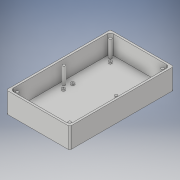
# Autodesk Inventor part: Box
Saved by Autodesk Inventor 2019 (Build 230136000, 136)
## iProperties
Created: 2018-10-23
Part Number: Box
Material: Generic
Document SubType Name: Modeling
Designer: Administrator
Density: 1 g/cm^3
Appearance: Default
Author: Administrator
Autodesk Inventor part; units mm, degrees
ref_plane "YZ Plane" through (0, 0, 0) normal (1, 0, 0) x (0, 1, 0)
ref_plane "XZ Plane" through (0, 0, 0) normal (0, 1, 0) x (-1, 0, 0)
ref_plane "XY Plane" through (0, 0, 0) normal (0, 0, 1) x (1, 0, 0)
sketch "Sketch1" plane through (0, 0, 0) normal (0, 1, 0) x (-1, 0, 0)
  line L0 (3.175, 0) -> (125.603, 0)
  line L1 (128.778, -3.175) -> (128.778, -208.153)
  line L2 (125.603, -211.328) -> (3.175, -211.328)
  line L3 (0, -208.153) -> (0, -3.175)
  line L4 (10.414, -4.064) -> (118.364, -4.064)
  line L5 (124.714, -10.414) -> (124.714, -200.914)
  line L6 (118.364, -207.264) -> (10.414, -207.264)
  line L7 (4.064, -200.914) -> (4.064, -10.414)
  circle A0 centre (117.348, -11.43) radius 2.794
  circle A1 centre (11.43, -11.43) radius 2.794
  circle A2 centre (117.348, -105.664) radius 2.794
  circle A3 centre (11.43, -105.664) radius 2.794
  circle A4 centre (117.348, -199.898) radius 2.794
  circle A5 centre (11.43, -199.898) radius 2.794
  line L8 (124.714, -105.664) -> (4.064, -105.664)
  line L9 (64.389, -4.064) -> (64.389, -207.264)
  circle A6 centre (108.839, -19.939) radius 1.143
  circle A7 centre (108.839, -19.939) radius 3.302
  circle A8 centre (108.839, -96.139) radius 3.302
  circle A9 centre (108.839, -96.139) radius 1.143
  circle A10 centre (19.939, -19.939) radius 3.302
  circle A11 centre (19.939, -19.939) radius 1.143
  circle A12 centre (19.939, -96.139) radius 3.302
  circle A13 centre (19.939, -96.139) radius 1.143
  circle A14 centre (108.839, -191.389) radius 1.143
  circle A15 centre (108.839, -191.389) radius 3.302
  circle A16 centre (108.839, -115.189) radius 3.302
  circle A17 centre (108.839, -115.189) radius 1.143
  circle A18 centre (19.939, -191.389) radius 3.302
  circle A19 centre (19.939, -191.389) radius 1.143
  circle A20 centre (19.939, -115.189) radius 3.302
  circle A21 centre (19.939, -115.189) radius 1.143
  arc A22 (128.778, -3.175) -> (125.603, 0) centre (125.603, -3.175) ccw
  arc A23 (125.603, -211.328) -> (128.778, -208.153) centre (125.603, -208.153) ccw
  arc A24 (0, -208.153) -> (3.175, -211.328) centre (3.175, -208.153) ccw
  arc A25 (3.175, 0) -> (0, -3.175) centre (3.175, -3.175) ccw
  arc A26 (10.414, -4.064) -> (4.064, -10.414) centre (10.414, -10.414) ccw
  arc A27 (124.714, -10.414) -> (118.364, -4.064) centre (118.364, -10.414) ccw
  arc A28 (118.364, -207.264) -> (124.714, -200.914) centre (118.364, -200.914) ccw
  arc A29 (4.064, -200.914) -> (10.414, -207.264) centre (10.414, -200.914) ccw
  point P0 (0, 0)
  point P1 (128.778, -211.328)
  point P2 (128.778, 0)
  point P3 (0, -211.328)
  dimension "d0" = 128.778
  dimension "d1" = 211.328
  dimension "d2" = 203.2
  dimension "d3" = 120.65
  dimension "d4" = 4.064
  dimension "d5" = 4.064
  dimension "d6" = 5.588
  dimension "d9" = 105.918
  dimension "d12" = 94.234
  dimension "d15" = 0
  dimension "d16" = 52.959
  dimension "d17" = 2.286
  dimension "d18" = 6.604
  dimension "d21" = 76.2
  dimension "d24" = 88.9
  dimension "d27" = 44.45
  dimension "d28" = 9.525
  dimension "d29" = 3.175
  dimension "d30" = 6.35
  dimension "d31" = 6.35
  constraints: 30 centre point, 20 end point, 16 point on circle, 16 tangent, 8 coincident, 8 point on line, 8 symmetric about line, 5 equal radius, 4 horizontal, 4 midpoint, 4 parallel, 2 perpendicular, 2 vertical, 30 other
  measures "d0" distance of point (128.778, -211.328) point (0, -211.328)
  measures "d1" distance of point (128.778, 0) point (128.778, -211.328)
  measures "d2" distance between parallel lines of L6 L4
  measures "d3" distance between parallel lines of L5 L7
  measures "d4" distance between parallel lines of L4 L0
  measures "d5" distance between parallel lines of L3 L7
  measures "d6" diameter of A0
  measures "d9" distance of A0.centre A1.centre
  measures "d12" distance of A0.centre A2.centre
  measures "d15" distance from line of L8 A2.centre
  measures "d16" distance from line of A0.centre L9
  measures "d17" diameter of A6
  measures "d18" diameter of A7
  measures "d21" distance of A7.centre A8.centre
  measures "d24" distance of A7.centre A10.centre
  measures "d27" distance from line of L9 A6.centre
  measures "d28" distance from line of L8 A8.centre
  measures "d29" radius of A22
  measures "d30" radius of A26
  measures "d31" radius of A27
extrude "Extrusion1" add sketch "Sketch1" along normal blind 3.556 contours L4 L9 L8 A3 L7 A26 | L4 A27 L5 L8 A2 L9 | L9 L6 A29 L7 L8 A3 | L8 A2 L5 A28 L6 L9
extrude "Extrusion2" add sketch "Sketch1" along normal blind 6.35 contours A7 | A8 | A10 | A12 | A15 | A16 | A18 | A20
extrude "Extrusion3" add sketch "Sketch1" along normal blind 38.1 contours L8 A2 | A2 L8 | L8 A3 | A3 L8 | A0 | A1 | A4 | A5
extrude "Extrusion4" add sketch "Sketch1" along normal blind 41.656 contours L0 A22 L1 A23 L2 A24 L3 A25
body "Solid1"
